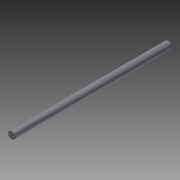
# Autodesk Inventor part: linear-guide-x
Saved by Autodesk Inventor 2012 (Build 160160000, 160)
## iProperties
Created: 2011-11-06
Part Number: linear-guide-x
Material: Galvanized Steel
Document SubType Name: Modeling
Designer: Aaron
Mass: 225.433 g
Surface Area: 97.7903 cm^2
Volume: 28.7176 cm^3
Density: 7.85 g/cm^3
Author: Aaron
Autodesk Inventor part; units mm, degrees
ref_plane "YZ Plane" through (0, 0, 0) normal (1, 0, 0) x (0, 1, 0)
ref_plane "XZ Plane" through (0, 0, 0) normal (0, 1, 0) x (-1, 0, 0)
ref_plane "XY Plane" through (0, 0, 0) normal (0, 0, 1) x (1, 0, 0)
sketch "Sketch1" plane through (0, 0, 0) normal (0, 0, 1) x (1, 0, 0)
  circle A0 centre (0, 0) radius 6
  dimension "d0" = 12
  constraints: 1 centre point, 1 coincident
  measures "d0" diameter of A0
extrude "Extrusion1" add sketch "Sketch1" along normal blind 254
chamfer "Chamfer1" distance 0.5 angle 45 2 edges at (-6, 0, 254) (-6, 0, 0)
body "Solid1"
